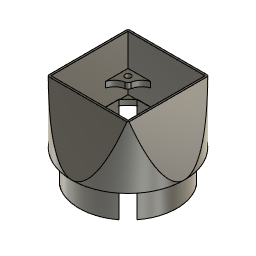
EPM_housing (Autodesk Fusion 360 design; units mm, degrees)
Autodesk Fusion 360 part; units mm, degrees
note: some values were not read from the file. Chosen so that the rebuilt part matches the saved one: which face or edge a step refers to. Set by a fixed rule: which sketch regions a step uses.
sketch "outer diameter" plane through (0, 0, 0) normal (0, 0, 1) x (1, 0, 0)
  circle A0 centre (0, 0) radius 29.79
  dimension "d1" = 59.58
  constraint coincident A0.centre origin
  measures "d1" diameter of A0
extrude "Extrude1" add sketch "outer diameter" along normal blind 47.8
sketch "inner diameter" plane through (0, 0, 0) normal (0, 0, -1) x (1, 0, 0)
  circle A0 centre (0, 0) radius 29.79
  circle A1 centre (0, 0) radius 25.79
  dimension "d4" = 51.58
  constraint coincident A0.centre A1.centre
  measures "d4" diameter of A1
extrude "Extrude2" cut sketch "inner diameter" against normal blind 15
sketch "o-ring" plane through (0, 0, 15) normal (0, 0, -1) x (1, 0, 0)
  circle A0 centre (0, 0) radius 25.79
  circle A1 centre (0, 0) radius 29.79
  circle A2 centre (0, 0) radius 28
  circle A3 centre (0, 0) radius 25.79
  constraint coincident A0.centre A1.centre
  constraint concentric A2 A3
extrude "Extrude3" cut sketch "o-ring" against normal blind 1 contours A2
sketch "inferior cavity" plane through (0, 0, 0) normal (0, 0, -1) x (1, 0, 0)
  circle A0 centre (0, 0) radius 25.79
  line L0 (20.45, 20.45) -> (-20.45, 20.45)
  line L1 (-20.45, 20.45) -> (-20.45, -20.45)
  line L2 (-20.45, -20.45) -> (20.45, -20.45)
  line L3 (20.45, -20.45) -> (20.45, 20.45)
  line L4 (20.45, 20.45) -> (-20.45, -20.45) construction
  line L5 (-20.45, 20.45) -> (20.45, -20.45) construction
  dimension "d9" = 40.9
  dimension "d10" = 40.9
  constraint horizontal L0
  constraint perpendicular L0 L1
  constraint parallel L0 L2
  constraint parallel L1 L3
  constraint coincident L4 A0.centre
  constraint coincident L5 A0.centre
  constraint coincident A0.centre origin
  measures "d9" distance of L1.end L2.end
  measures "d10" distance of L0.end L1.end
extrude "Extrude4" cut sketch "inferior cavity" against normal blind 19 contours A0 L0 L1 L2 L3
sketch "superior cavity" plane through (0, 0, 47.8) normal (0, 0, 1) x (-1, 0, 0)
  circle A0 centre (0, 0) radius 29.79
  line L0 (-20.35, -20.35) -> (20.35, -20.35)
  line L1 (20.35, -20.35) -> (20.35, 20.35)
  line L2 (20.35, 20.35) -> (-20.35, 20.35)
  line L3 (-20.35, 20.35) -> (-20.35, -20.35)
  line L4 (-20.35, -20.35) -> (20.35, 20.35) construction
  line L5 (20.35, -20.35) -> (-20.35, 20.35) construction
  line L6 (-21.35, -21.35) -> (21.35, -21.35)
  line L7 (21.35, -21.35) -> (21.35, 21.35)
  line L8 (21.35, 21.35) -> (-21.35, 21.35)
  line L9 (-21.35, 21.35) -> (-21.35, -21.35)
  line L10 (-21.35, -21.35) -> (21.35, 21.35) construction
  line L11 (21.35, -21.35) -> (-21.35, 21.35) construction
  dimension "d13" = 40.7
  dimension "d14" = 40.7
  dimension "d15" = 42.7
  dimension "d16" = 42.7
  constraint horizontal L0
  constraint perpendicular L0 L1
  constraint parallel L0 L2
  constraint parallel L1 L3
  constraint coincident L4 A0.centre
  constraint coincident L5 A0.centre
  constraint coincident A0.centre origin
  constraint horizontal L6
  constraint perpendicular L6 L7
  constraint parallel L6 L8
  constraint parallel L7 L9
  constraint coincident L10 A0.centre
  constraint coincident L11 A0.centre
  measures "d13" distance of L1.end L2.end
  measures "d14" distance of L0.end L1.end
  measures "d15" distance of L7.end L8.end
  measures "d16" distance of L6.end L7.end
extrude "Extrude5" cut sketch "superior cavity" against normal blind 29 contours L0 L1 L2 L3
ref_plane "WorkPlane1" through (0, 0, 30.8) normal (0, 0, 1) x (1, 0, 0)
sketch "mag mount" plane through (0, 0, 30.8) normal (0, 0, 1) x (1, 0, 0)
  line L0 (-20.35, 20.35) -> (-8.45, 20.35)
  line L1 (-20.35, 20.35) -> (-13.45, 20.35) construction
  line L2 (-13.45, 20.35) -> (-13.45, 13.45) construction
  line L3 (-20.35, 13.45) -> (-20.35, 20.35) construction
  line L4 (-20.35, 16.9) -> (-16.9, 16.9) construction
  circle A0 centre (-16.9, 16.9) radius 1.55 construction
  arc A1 (-8.45, 20.35) -> (-13.45, 13.45) centre (-6.189, 13.45) ccw
  line L5 (-20.35, 20.35) -> (-20.35, 13.45)
  line L6 (0, 20) -> (0, -20) construction
  line L7 (20.35, 20.35) -> (20.35, 13.45)
  line L8 (20.35, 20.35) -> (8.45, 20.35)
  arc A2 (13.45, 13.45) -> (8.45, 20.35) centre (6.189, 13.45) ccw
  line L9 (13.45, 13.45) -> (20.35, 13.45)
  circle A3 centre (16.9, 16.9) radius 1.55 construction
  line L10 (0, 0) -> (-12.0686, 0) construction
  arc A4 (-13.45, -13.45) -> (-8.45, -20.35) centre (-6.189, -13.45) ccw
  line L11 (-13.45, -13.45) -> (-20.35, -13.45) construction
  line L12 (-20.35, -20.35) -> (-20.35, -13.45)
  line L13 (-20.35, -20.35) -> (-8.45, -20.35)
  circle A5 centre (-16.9, -16.9) radius 1.55 construction
  arc A6 (8.45, -20.35) -> (13.45, -13.45) centre (6.189, -13.45) ccw
  line L14 (20.35, -20.35) -> (20.35, -13.45)
  line L15 (20.35, -20.35) -> (8.45, -20.35)
  circle A7 centre (16.9, -16.9) radius 1.55 construction
  line L16 (-20.35, -13.45) -> (-20.35, -8.45)
  line L17 (20.35, -13.45) -> (20.35, -8.45)
  arc A8 (-20.35, -8.45) -> (-13.45, -13.45) centre (-13.45, -6.189) ccw
  line L18 (13.45, -13.45) -> (20.35, -13.45)
  line L19 (-20.35, 13.45) -> (-20.35, 8.45)
  arc A9 (-13.45, 13.45) -> (-20.35, 8.45) centre (-13.45, 6.189) ccw
  point P0 (-20.35, 20.35)
  dimension "d20" = 11.9
  dimension "d22" = 6.9
  dimension "d23" = 6.9
  dimension "d25" = 3.45
  dimension "d26" = 3.1
  dimension "d27" = 5
  dimension "d28" = 5
  dimension "d46" = 5
  constraint horizontal L0
  constraint coincident P0 L0.start
  constraint horizontal L1
  constraint vertical L2
  constraint vertical L3
  constraint midpoint L3 L4.start
  constraint perpendicular L3 L4
  constraint coincident L4.end A0.centre
  constraint tangent L2 A1
  constraint vertical L6
  constraint symmetric P0 L6 L7.start
  constraint symmetric L0.end L6 L8.end
  constraint symmetric L2.end L6 A2.start
  constraint symmetric L3.start L6 L7.end
  constraint symmetric A0 L6 A3
  constraint symmetric A1 L6 A2
  constraint coincident L10.start origin
  constraint perpendicular L6 L10
  constraint symmetric P0 L10 L12.start
  constraint symmetric L0.end L10 A4.end
  constraint symmetric L2.end L10 A4.start
  constraint symmetric L3.start L10 L11.end
  constraint symmetric A0 L10 A5
  constraint symmetric A1 L10 A4
  constraint symmetric L7.start L10 L14.start
  constraint symmetric L7.end L10 L14.end
  constraint symmetric L8.end L10 A6.start
  constraint symmetric A2.start L10 A6.end
  constraint symmetric A2 L10 A6
  constraint symmetric A3 L10 A7
  constraint perpendicular L11 L16
  constraint tangent L11 A8
  measures "d20" distance of P0 L0.end
  measures "d22" distance of P0 L1.end
  measures "d23" distance of P0 L3.start
  measures "d25" distance of L4.start L4.end
  measures "d26" diameter of A0
  measures "d27" distance of L11.end L16.end
  measures "d28" distance of L14.end L17.end
  measures "d46" distance of L3.start L19.end
extrude "Extrude6" add sketch "mag mount" against normal blind 3
sketch "mag holes" plane through (0, 0, 30.8) normal (0, 0, 1) x (1, 0, 0)
  circle A0 centre (16.9, 16.9) radius 1.55
  line L0 (0, 20) -> (0, -20)
  circle A1 centre (-16.9, 16.9) radius 1.55
  line L1 (0, 0) -> (-12.0686, 0)
  circle A2 centre (16.9, -16.9) radius 1.55
  circle A3 centre (-16.9, -16.9) radius 1.55
  dimension "d31" = 3.1
  constraint symmetric A0 L0 A1
  constraint symmetric A0 L1 A2
  constraint symmetric A1 L1 A3
  measures "d31" diameter of A0
extrude "Extrude7" cut sketch "mag holes" against normal blind 4
fillet "Fillet1" radius 2 2 edges at (13.45, 13.45, 29.3) (-13.45, -13.45, 29.3)
sketch "side slants" plane through (0, 0, 0) normal (1, 0, 0) x (0, 1, 0)
  line L0 (-29.79, 15) -> (-21.35, 47.8)
  line L1 (-21.35, 47.8) -> (-29.79, 47.8)
  line L2 (-29.79, 47.8) -> (-29.79, 15)
  line L3 (0, 47.8) -> (0, 14) construction
  line L4 (21.35, 47.8) -> (29.79, 47.8)
  line L5 (29.79, 47.8) -> (29.79, 15)
  line L6 (29.79, 15) -> (21.35, 47.8)
  constraint horizontal L1
  constraint perpendicular L1 L2
  constraint vertical L3
  constraint symmetric L0.end L3 L4.start
  constraint symmetric L1.end L3 L4.end
  constraint symmetric L0.start L3 L5.end
extrude "Extrude8" cut sketch "side slants" along normal mid plane 60 contours L0 L1 L2
extrude "Extrude9" cut sketch "side slants" along normal mid plane 140 contours L4 L5 L6
sketch "side slants (1)" plane through (0, 0, 0) normal (0, 1, 0) x (1, 0, 0)
  line L0 (-29.79, -47.8) -> (-29.79, -15)
  line L1 (-29.79, -15) -> (-21.35, -47.8)
  line L2 (-21.35, -47.8) -> (-29.79, -47.8)
  line L3 (0, -49) -> (0, -36) construction
  line L4 (0, -47.8) -> (0, -15)
  line L5 (29.79, -15) -> (21.35, -47.8)
  line L6 (21.35, -47.8) -> (29.79, -47.8)
  line L7 (29.79, -47.8) -> (29.79, -15)
  constraint vertical L0
  constraint perpendicular L0 L2
  constraint vertical L3
  constraint symmetric L0.start L4 L6.end
  constraint symmetric L0.end L4 L5.start
  constraint symmetric L1.end L4 L5.end
extrude "Extrude10" cut sketch "side slants (1)" along normal mid plane 94
fillet "Fillet2" radius 2 2 edges at (-13.45, 13.45, 29.3) (13.45, -13.45, 29.3)
sketch "Sketch11" plane through (0, 0, 0) normal (0, 0, -1) x (1, 0, 0)
  line L0 (-15.7137, 20.45) -> (15.7137, 20.45)
  arc A0 (15.7137, 20.45) -> (-15.7137, 20.45) centre (0, 0) ccw
  line L1 (0, 20.45) -> (10.475, 20.45) construction
  line L2 (10.475, 20.45) -> (12.325, 20.45)
  line L3 (12.325, 20.45) -> (12.325, 22.13)
  line L4 (12.325, 22.13) -> (10.475, 22.13)
  line L5 (10.475, 22.13) -> (10.475, 20.45)
  line L6 (0, 0) -> (11, 0) construction
  line L7 (12.325, -22.13) -> (10.475, -22.13)
  line L8 (10.475, -22.13) -> (10.475, -20.45)
  line L9 (10.475, -20.45) -> (12.325, -20.45)
  line L10 (12.325, -20.45) -> (12.325, -22.13)
  dimension "d49" = 10.475
  dimension "d50" = 1.85
  dimension "d51" = 1.68
  constraint midpoint L0 L1.start
  constraint parallel L0 L1
  constraint horizontal L2
  constraint vertical L3
  constraint horizontal L4
  constraint vertical L5
  constraint coincident A0.centre L6.start
  constraint horizontal L6
  constraint symmetric L1.end L6 L8.end
  constraint symmetric L2.end L6 L9.end
  constraint symmetric L3.end L6 L7.start
  constraint symmetric L4.end L6 L7.end
  measures "d49" distance of L1.start L1.end
  measures "d50" distance of L1.end L2.end
  measures "d51" distance of L1.end L4.end
extrude "Extrude11" cut sketch "Sketch11" against normal blind 28 contours L0 L2 L3 L4 L5 | L7 L8 L9 L10
sketch "Sketch12" plane through (0, -22.13, 0) normal (0, 1, 0) x (-1, 0, 0)
  line L0 (-12.325, 0) -> (-10.475, 0)
  line L1 (-10.475, 0) -> (-10.475, 28)
  line L2 (-10.475, 28) -> (-12.325, 28)
  line L3 (-12.325, 28) -> (-12.325, 0)
  line L4 (-12.325, 0) -> (-10.475, 0)
  line L5 (-10.475, 0) -> (-10.475, 28.8624)
  line L6 (-10.475, 28.8624) -> (-12.325, 28.8624)
  line L7 (-12.325, 28.8624) -> (-12.325, 0)
  constraint perpendicular L4 L5
  constraint parallel L4 L6
  constraint parallel L5 L7
  constraint coincident L0.end L1.start
  constraint perpendicular L1 L4
  constraint coincident L0.start L3.end
extrude "Extrude12" cut sketch "Sketch12" along normal blind 43.5 contours L0 L1 L2 L3 L4 L5 L7
